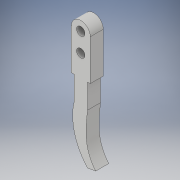
# Autodesk Inventor part: Abzug
Saved by Autodesk Inventor 2019 (Build 230136000, 136)
## iProperties
Created: 2021-03-08
Part Number: Abzug
Material: Generic
Document SubType Name: Modeling
Designer: Lukas
Density: 1 g/cm^3
Appearance: Default
Author: Lukas
Autodesk Inventor part; units mm, degrees
ref_plane "YZ Plane" through (0, 0, 0) normal (1, 0, 0) x (0, 1, 0)
ref_plane "XZ Plane" through (0, 0, 0) normal (0, 1, 0) x (-1, 0, 0)
ref_plane "XY Plane" through (0, 0, 0) normal (0, 0, 1) x (1, 0, 0)
sketch "Sketch1" plane through (0, 0, 0) normal (0, 0, 1) x (1, 0, 0)
  line L0 (-2.5, 0) -> (-2.5, -9)
  line L1 (2.5, 0) -> (2.5, -9)
  line L2 (-2.5, -9) -> (-3.5, -13) construction
  line L3 (-3.5, -13) -> (-3.5, -21) construction
  line L4 (-3.5, -21) -> (2.5, -27.5) construction
  spline S0 degree 3 poles (-2.5, -9) (-3.5, -13) (-3.5, -21) (2.5, -27.5) knots 1 1 1 1 2 2 2 2
  line L5 (2.5, -27.5) -> (5.5, -27)
  line L6 (5.5, -27) -> (1.5, -22) construction
  line L7 (1.5, -22) -> (1.5, -17) construction
  line L8 (1.5, -17) -> (2.5, -9) construction
  spline S1 degree 3 poles (5.5, -27) (1.5, -22) (1.5, -17) (2.5, -9) knots 1 1 1 1 2 2 2 2
  line L9 (2.5, 0) -> (3.5, 0)
  line L10 (3.5, 0) -> (3.5, 15)
  line L11 (-3.5, 15) -> (-3.5, 0)
  line L12 (-3.5, 0) -> (-2.5, 0)
  circle A0 centre (0, 15) radius 1.55
  arc A1 (3.5, 15) -> (-3.5, 15) centre (0, 15) ccw
  circle A2 centre (0, 8) radius 1.55
  point P0 (0, 0)
  dimension "d8" = 1
  dimension "d9" = 3
  dimension "d10" = 3
  dimension "d11" = 18
  dimension "d12" = 8
  dimension "d13" = 5
  dimension "d15" = 0.5
  dimension "d17" = 1
  dimension "d18" = 4
  dimension "d19" = 8
  dimension "d25" = 5
  dimension "d26" = 2.5
  dimension "d27" = 9
  dimension "d29" = 1
  dimension "d30" = 1
  dimension "d44" = 3.1
  dimension "d45" = 7
  dimension "d47" = 24
  constraints: 14 end point, 3 centre point, 3 vertical, 3 vertical alignment, 2 horizontal alignment, 2 perpendicular, 2 point on circle, 2 tangent, 1 coincident, 1 equal radius, 1 horizontal, 1 parallel, 1 point on line, 6 other
  measures "d8" distance from line of L1 L7.end
  measures "d9" distance from line of L1 L5.end
  measures "d10" horizontal distance of L5.end L4.end
  measures "d11" vertical distance of L1.end L5.end
  measures "d12" vertical distance of L1.end L7.end
  measures "d13" distance of L7.end L6.end
  measures "d15" vertical distance of L5.end L4.end
  measures "d17" distance from line of L0 L2.end
  measures "d18" vertical distance of L0.end L2.end
  measures "d19" distance of L3.end L2.end
  measures "d25" distance between parallel lines of L0 L1
  measures "d26" distance from line of point (0, 0) L1
  measures "d27" distance of L0.start L0.end
  measures "d29" distance of L1.start L9.end
  measures "d30" distance of L11.end L0.start
  measures "d44" diameter of A0
  measures "d45" distance of A0.centre A2.centre
  measures "d47" vertical distance of L1.end A0.centre
extrude "Extrusion1" add sketch "Sketch1" along normal blind 4.8
equation "\"d26\" = 0.5 * d25"
body "Solid1"
